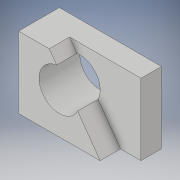
# Autodesk Inventor part: Part6
Saved by Autodesk Inventor 2017 (Build 210142000, 142)
## iProperties
Created: 2016-11-03
Part Number: Part6
Material: Generic
Document SubType Name: Modeling
Designer: s411888
Density: 1 g/cm^3
Appearance: Default
Author: s411888
Autodesk Inventor part; units mm, degrees
ref_plane "YZ Plane" through (0, 0, 0) normal (1, 0, 0) x (0, 1, 0)
ref_plane "XZ Plane" through (0, 0, 0) normal (0, 1, 0) x (-1, 0, 0)
ref_plane "XY Plane" through (0, 0, 0) normal (0, 0, 1) x (1, 0, 0)
sketch "Sketch1" plane through (0, 0, 0) normal (0, 0, 1) x (1, 0, 0)
  line L0 (-29.5214, 15.9367) -> (33.9786, 15.9367)
  line L1 (33.9786, 15.9367) -> (33.9786, -28.5133)
  line L2 (33.9786, -28.5133) -> (-29.5214, -28.5133)
  line L3 (-29.5214, -28.5133) -> (-29.5214, 15.9367)
  point P0 (0, 0)
  dimension "d0" = 63.5
  dimension "d1" = 44.45
  constraints: 8 end point, 2 parallel, 1 horizontal, 1 perpendicular
  measures "d0" distance of L1.end L2.end
  measures "d1" distance of L0.end L1.end
extrude "Extrusion1" add sketch "Sketch1" along normal blind 25.4
sketch "Sketch2" plane through (0, 0, 25.4) normal (0, 0, 1) x (1, 0, 0)
  line L0 (33.9786, 15.9367) -> (-29.5214, 15.9367) projected
  line L1 (-29.5214, -28.5133) -> (33.9786, -28.5133) projected
  line L2 (-10.4714, 15.9367) -> (33.9786, 15.9367)
  line L3 (33.9786, 15.9367) -> (33.9786, -28.5133)
  line L4 (-10.4714, 15.9367) -> (21.2786, -28.5133)
  point P0 (0, 0)
  dimension "d4" = 19.05
  dimension "d12" = 12.7
  constraints: 6 end point, 2 point on line, 1 vertical
  measures "d4" distance of L0.end L2.start
  measures "d12" distance of L1.end L4.end
extrude "Extrusion2" cut sketch "Sketch2" against normal blind 12.7
sketch "Sketch3" plane through (0, 0, 25.4) normal (0, 0, 1) x (1, 0, 0)
  line L0 (33.9786, -28.5133) -> (-29.5214, -28.5133) projected
  line L1 (33.9786, -28.5133) -> (8.5786, -28.5133)
  circle A0 centre (-4.1214, -3.1133) radius 12.7
  line L2 (-29.5214, 15.9367) -> (-29.5214, -28.5133) projected
  point P0 (0, 0)
  dimension "d14" = 25.4
  dimension "d15" = 25.4
  dimension "d16" = 25.4
  constraints: 2 end point, 1 centre point, 1 horizontal
  measures "d14" diameter of A0
  measures "d15" distance from line of L2 A0.centre
  measures "d16" distance from line of L0 A0.centre
extrude "Extrusion3" cut sketch "Sketch3" against normal blind 25.4
body "Solid1"
